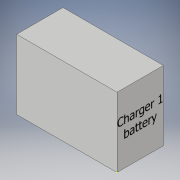
# Autodesk Inventor part: 1 battery charger 2019
Saved by Autodesk Inventor 2019 (Build 230136000, 136)
## iProperties
Created: 2018-12-09
Part Number: 1 battery charger 2019
Material: Generic
Document SubType Name: Modeling
Designer: Tiberus
Density: 1 g/cm^3
Appearance: Default
Author: Tiberus
Autodesk Inventor part; units mm, degrees
ref_plane "YZ Plane" through (0, 0, 0) normal (1, 0, 0) x (0, 1, 0)
ref_plane "XZ Plane" through (0, 0, 0) normal (0, 1, 0) x (-1, 0, 0)
ref_plane "XY Plane" through (0, 0, 0) normal (0, 0, 1) x (1, 0, 0)
sketch "Sketch1" plane through (0, 0, 0) normal (0, 1, 0) x (-1, 0, 0)
  line L0 (0, 0) -> (165.1, 0)
  line L1 (165.1, 0) -> (165.1, -76.2)
  line L2 (165.1, -76.2) -> (0, -76.2)
  line L3 (0, -76.2) -> (0, 0)
  dimension "d0" = 165.1
  dimension "d1" = 76.2
  constraints: 8 end point, 2 parallel, 1 horizontal, 1 perpendicular
  measures "d0" distance of L1.end L2.end
  measures "d1" distance of L0.end L1.end
extrude "Extrusion1" add sketch "Sketch1" along normal blind 114.3
sketch "Sketch2" plane through (0, 0, 0) normal (1, 0, 0) x (0, 0, -1)
  line L0 (0, 114.3818) -> (76.3652, 114.3818) construction
  line L1 (76.3652, 114.3818) -> (76.3652, 0) construction
  line L2 (76.3652, 0) -> (0, 0) construction
  line L3 (0, 0) -> (0, 114.3818) construction
  point P0 (0, 0)
  constraints: 2 other
body "Solid1"
